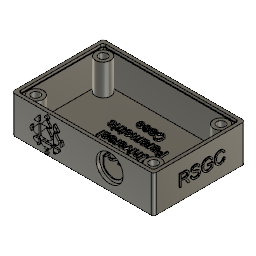
ACESUniversalST1StripboardCase v4 (Autodesk Fusion 360 design; units mm, degrees)
Autodesk Fusion 360 part; units mm, degrees
note: some values were not read from the file. Set by a fixed rule: which sketch regions a step uses.
sketch "PCB" plane through (0, 0, 0) normal (0, 0, 1) x (1, 0, 0)
  line L0 (0, 0) -> (80, 0)
  line L1 (80, 0) -> (80, 50)
  line L2 (80, 50) -> (0, 50)
  line L3 (0, 50) -> (0, 0)
  line L4 (-0.25, -0.25) -> (80.25, -0.25)
  line L5 (80.25, -0.25) -> (80.25, 50.25)
  line L6 (80.25, 50.25) -> (-0.25, 50.25)
  line L7 (-0.25, 50.25) -> (-0.25, -0.25)
  line L8 (79.75, 0.25) -> (79.75, 49.75)
  line L9 (79.75, 49.75) -> (0.25, 49.75)
  line L10 (0.25, 49.75) -> (0.25, 0.25)
  line L11 (0.25, 0.25) -> (79.75, 0.25)
  line L12 (82.25, 52.25) -> (-2.25, 52.25)
  line L13 (-2.25, 52.25) -> (-2.25, -2.25)
  line L14 (-2.25, -2.25) -> (82.25, -2.25)
  line L15 (82.25, -2.25) -> (82.25, 52.25)
  dimension "d7" = 80
  dimension "d8" = 50
  dimension "d30" = 0.25
  dimension "d32" = 2.25
  constraint horizontal L0
  constraint vertical L1
  constraint horizontal L2
  constraint vertical L3
  constraint coincident L0.start L3.end
  measures "d7" distance of L0.start L0.end
  measures "d8" distance of L0.start L2.end
sketch "Piers" plane through (0, 0, 0) normal (0, 0, 1) x (1, 0, 0)
  line L0 (80, 50) -> (0, 50)
  circle A0 centre (5, 45) radius 4.5
  circle A1 centre (5, 45) radius 2.5
  line L1 (0, 50) -> (0, 0)
  line L2 (0, 0) -> (80, 0)
  circle A2 centre (5, 5) radius 4.5
  circle A3 centre (5, 5) radius 2.5
  line L3 (80, 0) -> (80, 50)
  circle A4 centre (75, 45) radius 4.5
  circle A5 centre (75, 45) radius 2.5
  circle A6 centre (75, 5) radius 4.5
  circle A7 centre (75, 5) radius 2.5
  point P0 (5, 45)
  point P1 (0, 50)
  point P2 (5, 5)
  point P3 (75, 45)
  point P4 (75, 5)
  point P5 (75, 5)
  dimension "d10" = 5
  dimension "d11" = 5
  dimension "d13" = 9
  dimension "d15" = 5
  dimension "d16" = 5
  dimension "d17" = 5
  dimension "d18" = 9
  dimension "d19" = 5
  dimension "d20" = 5
  dimension "d21" = 5
  dimension "d22" = 9
  dimension "d23" = 5
  dimension "d24" = 5
  dimension "d25" = 5
  dimension "d26" = 9
  dimension "d27" = 5
  constraint coincident P0 A0.centre
  constraint coincident P2 A2.centre
  constraint coincident P3 A4.centre
  constraint coincident P5 P4
  constraint concentric A6 A7
  measures "d10" horizontal distance of P0 L0.end
  measures "d11" distance of P0 L0
  measures "d13" diameter of A0
  measures "d15" diameter of A1
  measures "d16" distance of P2 L1
  measures "d17" distance of P2 L2
  measures "d18" diameter of A2
  measures "d19" diameter of A3
  measures "d20" distance of P3 L3
  measures "d21" distance of L0 P3
  measures "d22" diameter of A4
  measures "d23" diameter of A5
  measures "d24" distance of L3 P5
  measures "d25" distance of L2 P5
  measures "d26" diameter of A6
  measures "d27" diameter of A7
extrude "Extrude1" add sketch "Piers" along normal blind 20.4 contours A4 makes body 1
extrude "Extrude2" add sketch "Piers" along normal blind 13 contours A5 bodies 1
extrude "Extrude3" add sketch "Piers" along normal blind 13 separate body contours A7 makes body 2
extrude "Extrude4" add sketch "Piers" along normal blind 20.4 contours A6 bodies 2
extrude "Extrude5" add sketch "Piers" along normal blind 13 separate body contours A3 makes body 3
extrude "Extrude6" add sketch "Piers" along normal blind 20.4 contours A2 bodies 3
extrude "Extrude7" add sketch "Piers" along normal blind 13 separate body contours A1 makes body 4
extrude "Extrude8" add sketch "Piers" along normal blind 20.4 contours A0 bodies 4
extrude "Extrude9" cut sketch "PCB" along normal blind 2 contours L8 L9 L10 L11 bodies 1 2 3 4
extrude "Extrude10" add sketch "PCB" along normal blind 2 contours L8 L9 L10 L11 bodies 1 2 3 4
extrude "Extrude11" add sketch "PCB" along normal blind 20.4 contours L0 L1 L2 L3 bodies 1
extrude "Extrude12" add sketch "PCB" along normal blind 20.4 contours L4 L5 L6 L7 bodies 1
extrude "Extrude13" add sketch "PCB" along normal blind 22 contours L12 L13 L14 L15 bodies 1
fillet "Fillet1" radius 1.5 4 edges at (82.25, -2.25, 11) (-2.25, -2.25, 11) (82.25, 52.25, 11) (-2.25, 52.25, 11) on bodies 1
fillet "Fillet2" radius 1.5 1 edges at (80.25, -0.25, 21.2) on bodies 1
fillet "Fillet3" radius 1.5 1 edges at (-0.25, 50.25, 21.2) on bodies 1
fillet "Fillet4" radius 1.5 1 edges at (-0.25, -0.25, 21.2) on bodies 1
fillet "Fillet5" radius 1.5 1 edges at (80.25, 50.25, 21.2) on bodies 1
sketch "SchurterPJ" plane through (0, -2.25, 0) normal (0, -1, 0) x (1, 0, 0)
  line L0 (-0.75, 22) -> (-0.75, 0)
  line L1 (-0.75, 0) -> (80.75, 0)
  line L2 (80.75, 0) -> (80.75, 22)
  line L3 (80.75, 22) -> (-0.75, 22)
  circle A0 centre (56.0888, 11.8801) radius 8
  circle A1 centre (56.0888, 11.8801) radius 6.4
  line L4 (50.1888, 9.4002) -> (50.1888, 14.36)
  line L5 (61.9888, 14.36) -> (61.9888, 9.4002)
  line L6 (61.9888, 9.4002) -> (50.1888, 14.36) construction
  line L7 (50.1888, 9.4002) -> (61.9888, 14.36) construction
  point P0 (56.0888, 11.8801)
  dimension "d84" = 16
  dimension "d85" = 12.8
  dimension "d86" = 11.8
  constraint concentric A0 A1
  constraint parallel L4 L5
  constraint coincident L6 P0
  constraint coincident L7 P0
  constraint coincident A1 L5.end
  constraint coincident P0 A0.centre
  measures "d84" diameter of A0
  measures "d85" diameter of A1
  measures "d86" distance of L4.end L5.start
extrude "Extrude16" cut sketch "SchurterPJ" against normal blind 4 contours A1 L4 L5 bodies 1
extrude "Extrude17" cut sketch "SchurterPJ" against normal blind 2 contours A0 bodies 1
extrude "Extrude18" cut sketch "SchurterPJ" against normal blind 2 contours A1 L4 bodies 1
extrude "Extrude19" cut sketch "SchurterPJ" against normal blind 2 contours A1 L5 bodies 1
sketch "RSGC" plane through (82.25, 0, 0) normal (1, 0, 0) x (0, 1, 0)
  line L0 (50.75, 0) -> (50.75, 22)
  line L1 (50.75, 22) -> (-0.75, 22)
  line L2 (-0.75, 22) -> (-0.75, 0)
  line L3 (-0.75, 0) -> (50.75, 0)
  line L4 (6.6478, 4.3711) -> (45.8969, 4.3711) construction
  line L5 (45.8969, 4.3711) -> (45.8969, 17.8488) construction
  line L6 (45.8969, 17.8488) -> (6.6478, 17.8488) construction
  line L7 (6.6478, 17.8488) -> (6.6478, 4.3711) construction
  dimension "d101" = 7
  text T0 "RSGC" font "Arial" height 7 align centre middle in box 39.2491 x 13.4777 at (6.6478, 4.3711) x (1, 0) y (0, 1) spacing 1
extrude "Extrude23" add sketch "RSGC" along normal blind 0.5 text T0 bodies 1
sketch "ACES" plane through (-2.25, 0, 0) normal (-1, 0, 0) x (0, -1, 0)
  line L0 (-50.75, 22) -> (-50.75, 0)
  line L1 (-50.75, 0) -> (0.75, 0)
  line L2 (0.75, 0) -> (0.75, 22)
  line L3 (0.75, 22) -> (-50.75, 22)
  line L4 (-44.8392, 4.4236) -> (-4.5213, 4.4236) construction
  line L5 (-4.5213, 4.4236) -> (-4.5213, 18.3404) construction
  line L6 (-4.5213, 18.3404) -> (-44.8392, 18.3404) construction
  line L7 (-44.8392, 18.3404) -> (-44.8392, 4.4236) construction
  dimension "d105" = 7
  text T0 "ACES" font "Arial" height 7 align centre middle in box 40.3179 x 13.9168 at (-44.8392, 4.4236) x (1, 0) y (0, 1) spacing 1
extrude "Extrude24" add sketch "ACES" along normal blind 0.5 text T0 bodies 1
sketch "Stripboard" plane through (0, 52.25, 0) normal (0, 1, 0) x (-1, 0, 0)
  line L0 (0.75, 0) -> (0.75, 22)
  line L1 (0.75, 22) -> (-80.75, 22)
  line L2 (-80.75, 22) -> (-80.75, 0)
  line L3 (-80.75, 0) -> (0.75, 0)
  line L4 (-75.2707, 4.2089) -> (-2.7407, 4.2089) construction
  line L5 (-2.7407, 4.2089) -> (-2.7407, 18.6953) construction
  line L6 (-2.7407, 18.6953) -> (-75.2707, 18.6953) construction
  line L7 (-75.2707, 18.6953) -> (-75.2707, 4.2089) construction
  dimension "d108" = 7
  text T0 "Stripboard" font "Arial" height 7 align centre middle in box 72.53 x 14.4864 at (-75.2707, 4.2089) x (1, 0) y (0, 1) spacing 1
extrude "Extrude25" add sketch "Stripboard" along normal blind 0.5 text T0 bodies 1
sketch "ACESLogo" plane through (0, -2.25, 0) normal (0, -1, 0) x (1, 0, 0)
  line L0 (-0.75, 22) -> (-0.75, 0)
  line L1 (-0.75, 0) -> (80.75, 0)
  line L2 (80.75, 0) -> (80.75, 22)
  line L3 (80.75, 22) -> (-0.75, 22)
  circle A0 centre (56.0888, 11.8801) radius 8
  arc A1 (18.9448, 9.0125) -> (17.9359, 8.8538) centre (17.8817, 12.4835) cw
  spline S0 degree 3 poles (17.9359, 8.8538) (17.1335, 8.9002) (16.4759, 9.5075) (16.366, 10.3037) knots 1 1 1 1 2 2 2 2
  arc A2 (16.366, 10.3037) -> (16.8211, 11.6936) centre (18.2653, 10.4513) cw
  spline S1 degree 3 poles (16.8211, 11.6936) (17.5549, 12.5932) (18.2992, 13.4857) (19.033, 14.3889) knots 3 3 3 3 4 4 4 4
  spline S2 degree 3 poles (19.033, 14.3889) (19.193, 14.597) (19.4912, 14.6364) (19.6997, 14.4771) knots 4 4 4 4 5 5 5 5
  arc A3 (19.6997, 14.4771) -> (19.7879, 14.3889) centre (19.4528, 14.1419) cw
  spline S3 degree 3 poles (19.7879, 14.3889) (20.2289, 13.8279) (20.6981, 13.2952) (21.1497, 12.7449) knots 6 6 6 6 7 7 7 7
  arc A4 (21.1497, 12.7449) -> (22.1657, 11.482) centre (10.8021, 3.3805) cw
  spline S4 degree 3 poles (22.1657, 11.482) (22.695, 10.7422) (22.5262, 9.7137) (21.7882, 9.1819) knots 8 8 8 8 9 9 9 9
  arc A5 (21.7882, 9.1819) -> (21.2026, 8.9173) centre (20.8109, 10.5647) cw
  arc A6 (21.2026, 8.9173) -> (20.0702, 8.9737) centre (20.7508, 11.2409) cw
  spline S5 degree 3 poles (20.0702, 8.9737) (20.0067, 8.9737) (19.922, 9.0549) (19.8373, 8.949) (19.9044, 8.8749) (19.9255, 8.8114) knots 11 11 11 11 12 12 13 13 13 13
  arc A7 (19.9255, 8.8114) -> (20.2889, 8.1659) centre (23.5074, 10.4024) ccw
  spline S6 degree 3 poles (20.2889, 8.1659) (20.3348, 8.0953) (20.3947, 8.0212) (20.2889, 7.8378) (20.2007, 7.8554) (20.1125, 7.8554) knots 14 14 14 14 15 15 16 16 16 16
  line L4 (20.1125, 7.8554) -> (18.7014, 7.8554)
  arc A8 (18.7014, 7.8554) -> (18.5215, 7.9366) centre (18.6835, 8.0557) cw
  spline S7 degree 3 poles (18.5215, 7.9366) (18.4721, 8.0106) (18.5215, 8.0706) (18.5497, 8.1306) knots 18 18 18 18 19 19 19 19
  arc A9 (18.5497, 8.1306) -> (18.9448, 9.0125) centre (16.2293, 9.6996) ccw
  arc A10 (19.862, 4.8674) -> (20.2501, 4.0101) centre (22.6563, 5.6158) ccw
  arc A11 (20.2501, 4.0101) -> (20.3171, 3.9114) centre (19.4824, 3.4171) cw
  spline S8 degree 3 poles (20.3171, 3.9114) (20.3585, 3.843) (20.3367, 3.7541) (20.2684, 3.7127) knots 2 2 2 2 3 3 3 3
  spline S9 degree 3 poles (20.2684, 3.7127) (20.267, 3.7119) (20.2656, 3.7111) (20.2642, 3.7103) knots 3 3 3 3 4 4 4 4
  arc A12 (20.2642, 3.7103) -> (20.1795, 3.6891) centre (20.1938, 3.8118) cw
  line L5 (20.1795, 3.6891) -> (18.6308, 3.6891)
  spline S10 degree 3 poles (18.6308, 3.6891) (18.4862, 3.6891) (18.4297, 3.802) (18.5074, 3.929) knots 6 6 6 6 7 7 7 7
  arc A13 (18.5074, 3.929) -> (18.9025, 4.7016) centre (15.4234, 5.9935) ccw
  spline S11 degree 3 poles (18.9025, 4.7016) (18.9201, 4.751) (18.9519, 4.8074) (18.8531, 4.878) (18.8213, 4.8427) (18.779, 4.8215) knots 8 8 8 8 9 9 10 10 10 10
  arc A14 (18.779, 4.8215) -> (17.3467, 4.8427) centre (18.0946, 6.9768) cw
  spline S12 degree 3 poles (17.3467, 4.8427) (16.7529, 5.0971) (16.3626, 5.675) (16.3484, 6.3208) knots 11 11 11 11 12 12 12 12
  arc A15 (16.3484, 6.3208) -> (16.4083, 6.8077) centre (18.2321, 6.3359) cw
  spline S13 degree 3 poles (16.4083, 6.8077) (16.4227, 6.8898) (16.4982, 6.9469) (16.5812, 6.9382) knots 13 13 13 13 14 14 14 14
  line L6 (16.5812, 6.9382) -> (22.1445, 6.9382)
  spline S14 degree 3 poles (22.1445, 6.9382) (22.3032, 6.9382) (22.3738, 6.8853) (22.4056, 6.7406) knots 15 15 15 15 16 16 16 16
  spline S15 degree 3 poles (22.4056, 6.7406) (22.6249, 5.8696) (22.0966, 4.9858) (21.2256, 4.7664) knots 16 16 16 16 17 17 17 17
  line L7 (21.2256, 4.7664) -> (21.2202, 4.7651)
  line L8 (21.2202, 4.7651) -> (21.1673, 4.7651)
  arc A16 (21.1673, 4.7651) -> (19.862, 4.8674) centre (20.7187, 7.4191) cw
  spline S16 degree 3 poles (14.5139, 9.0125) (14.2846, 8.9561) (14.0659, 8.9102) (13.8472, 8.8749) knots 0 0 0 0 1 1 1 1
  spline S17 degree 3 poles (13.8472, 8.8749) (12.9414, 8.7275) (12.0877, 9.3423) (11.9402, 10.248) (11.8627, 10.7242) (11.9961, 11.2106) (12.3055, 11.5808) knots 1 1 1 1 2 2 2 3 3 3 3
  spline S18 degree 3 poles (12.3055, 11.5808) (12.7394, 12.1417) (13.2016, 12.6779) (13.6461, 13.2247) knots 3 3 3 3 4 4 4 4
  line L9 (13.6461, 13.2247) -> (14.6056, 14.3959)
  arc A17 (14.6056, 14.3959) -> (14.9584, 14.5723) centre (14.9478, 14.1526) cw
  spline S19 degree 3 poles (14.9584, 14.5723) (15.046, 14.5763) (15.1202, 14.5085) (15.1242, 14.4209) knots 6 6 6 6 7 7 7 7
  line L10 (15.1242, 14.4209) -> (15.1242, 14.4206)
  line L11 (15.1242, 14.4206) -> (15.1242, 8.0142)
  spline S20 degree 3 poles (15.1242, 8.0142) (15.144, 7.9237) (15.0874, 7.8341) (14.9972, 7.8131) knots 9 9 9 9 10 10 10 10
  line L12 (14.9972, 7.8131) -> (14.2423, 7.8131)
  arc A18 (14.2423, 7.8131) -> (14.0518, 7.9083) centre (14.2177, 8.002) cw
  spline S21 degree 3 poles (14.0518, 7.9083) (14.0059, 7.9754) (14.0518, 8.0318) (14.0871, 8.0847) knots 12 12 12 12 13 13 13 13
  arc A19 (14.0871, 8.0847) -> (14.5139, 9.0125) centre (11.5121, 9.8315) ccw
  line L13 (23.7002, 11.2068) -> (23.7002, 14.3077)
  spline S22 degree 3 poles (23.7002, 14.3077) (23.7002, 14.3994) (23.6614, 14.5159) (23.7814, 14.5582) knots 1 1 1 1 2 2 2 2
  arc A20 (23.7814, 14.5582) -> (24.1059, 14.4876) centre (23.8827, 14.2424) cw
  arc A21 (24.1059, 14.4876) -> (24.4305, 14.1102) centre (22.3461, 12.6463) cw
  spline S23 degree 3 poles (24.4305, 14.1102) (25.1184, 13.2811) (25.8169, 12.4556) (26.4837, 11.609) knots 4 4 4 4 5 5 5 5
  spline S24 degree 3 poles (26.4837, 11.609) (27.0909, 10.9209) (27.0253, 9.8709) (26.3372, 9.2637) (25.9609, 8.9316) (25.4545, 8.7874) (24.9597, 8.8714) knots 5 5 5 5 6 6 6 7 7 7 7
  spline S25 degree 3 poles (24.9597, 8.8714) (24.7692, 8.8996) (24.5857, 8.9314) (24.3988, 8.9772) knots 7 7 7 7 8 8 8 8
  spline S26 degree 3 poles (24.3988, 8.9772) (24.3705, 8.9772) (24.3458, 9.0161) (24.2894, 8.9384) (24.3176, 8.9243) (24.3176, 8.8926) knots 8 8 8 8 9 9 10 10 10 10
  arc A22 (24.3176, 8.8926) -> (24.6457, 8.187) centre (27.442, 9.9164) ccw
  spline S27 degree 3 poles (24.6457, 8.187) (24.7021, 8.0882) (24.815, 7.9965) (24.681, 7.7496) (24.5399, 7.8025) (24.4305, 7.799) knots 11 11 11 11 12 12 13 13 13 13
  line L14 (24.4305, 7.799) -> (23.9013, 7.799)
  spline S28 degree 3 poles (23.9013, 7.799) (23.7249, 7.799) (23.6967, 7.8342) (23.6967, 8.0001) knots 14 14 14 14 15 15 15 15
  line L15 (23.6967, 8.0001) -> (23.7002, 11.2068)
  line L16 (21.8023, 15.5036) -> (20.4723, 15.5036)
  spline S29 degree 3 poles (20.4723, 15.5036) (19.9679, 15.5036) (19.4599, 15.4789) (18.9554, 15.5036) knots 1 1 1 1 2 2 2 2
  line L17 (18.9554, 15.5036) -> (16.8952, 15.5036)
  arc A23 (16.8952, 15.5036) -> (16.7223, 15.5918) centre (16.8776, 15.6827) cw
  ellipse E0 centre (16.8568, 15.657) end of major axis (16.8885, 15.804) minor radius 0.1488 (16.7611, 15.7717) -> (16.7223, 15.5918) ccw
  arc A24 (16.7611, 15.7717) -> (19.033, 18.5305) centre (514.2406, -391.6025) cw
  spline S30 degree 3 poles (19.033, 18.5305) (19.1707, 18.7375) (19.4498, 18.7943) (19.6574, 18.6575) knots 6 6 6 6 7 7 7 7
  arc A25 (19.6574, 18.6575) -> (19.7985, 18.5093) centre (19.42, 18.2901) cw
  spline S31 degree 3 poles (19.7985, 18.5093) (20.1125, 18.1177) (20.4406, 17.7367) (20.7616, 17.3487) knots 8 8 8 8 9 9 9 9
  line L18 (20.7616, 17.3487) -> (21.8199, 16.054)
  spline S32 degree 3 poles (21.8199, 16.054) (21.8976, 15.9587) (21.9716, 15.8635) (22.0528, 15.7753) knots 10 10 10 10 11 11 11 11
  ellipse E1 centre (21.9602, 15.6624) end of major axis (21.9286, 15.8059) minor radius 0.1453 (22.0916, 15.5989) -> (22.0528, 15.7753) ccw
  spline S33 degree 3 poles (22.0916, 15.5989) (22.0643, 15.5318) (21.9934, 15.4934) (21.9223, 15.5072) knots 12 12 12 12 13 13 13 13
  arc A26 (21.9223, 15.5072) -> (21.8023, 15.5036) centre (21.8725, 15.1579) ccw
  arc A27 (24.3423, 4.8603) -> (24.748, 3.9996) centre (27.4138, 5.782) ccw
  spline S34 degree 3 poles (24.748, 3.9996) (24.7903, 3.9325) (24.8397, 3.869) (24.748, 3.6926) (24.6669, 3.7138) (24.5963, 3.7138) knots 1 1 1 1 2 2 3 3 3 3
  line L19 (24.5963, 3.7138) -> (23.919, 3.7138)
  spline S35 degree 3 poles (23.919, 3.7138) (23.7849, 3.7138) (23.732, 3.7703) (23.732, 3.9043) knots 4 4 4 4 5 5 5 5
  line L20 (23.732, 3.9043) -> (23.732, 6.7547)
  spline S36 degree 3 poles (23.732, 6.7547) (23.732, 6.8853) (23.7884, 6.9523) (23.919, 6.9523) knots 6 6 6 6 7 7 7 7
  line L21 (23.919, 6.9523) -> (26.6848, 6.9523)
  spline S37 degree 3 poles (26.6848, 6.9523) (26.7676, 6.9636) (26.8454, 6.9102) (26.8647, 6.8288) knots 8 8 8 8 9 9 9 9
  spline S38 degree 3 poles (26.8647, 6.8288) (27.1112, 5.957) (26.6043, 5.0505) (25.7325, 4.804) knots 9 9 9 9 10 10 10 10
  line L22 (25.7325, 4.804) -> (25.7323, 4.8039)
  arc A28 (25.7323, 4.8039) -> (25.5029, 4.758) centre (25.2724, 6.5069) cw
  arc A29 (25.5029, 4.758) -> (24.4446, 4.878) centre (25.2859, 7.5719) cw
  line L23 (24.4446, 4.878) -> (24.3846, 4.878)
  line L24 (24.3846, 4.878) -> (24.3423, 4.8603)
  arc A30 (14.5104, 4.8639) -> (13.5226, 4.7192) centre (13.4801, 8.4549) cw
  spline S39 degree 3 poles (13.5226, 4.7192) (12.9343, 4.7273) (12.3955, 5.0506) (12.1115, 5.5659) knots 1 1 1 1 2 2 2 2
  arc A31 (12.1115, 5.5659) -> (11.9669, 6.7547) centre (13.4646, 6.3337) cw
  spline S40 degree 3 poles (11.9669, 6.7547) (11.9862, 6.8526) (12.0755, 6.9207) (12.175, 6.9135) knots 3 3 3 3 4 4 4 4
  line L25 (12.175, 6.9135) -> (14.8949, 6.9135)
  spline S41 degree 3 poles (14.8949, 6.9135) (15.0748, 6.9135) (15.1066, 6.8747) (15.1066, 6.6877) knots 5 5 5 5 6 6 6 6
  line L26 (15.1066, 6.6877) -> (15.1066, 3.8973)
  spline S42 degree 3 poles (15.1066, 3.8973) (15.1066, 3.7456) (15.0572, 3.6891) (14.902, 3.6891) knots 7 7 7 7 8 8 8 8
  line L27 (14.902, 3.6891) -> (14.2493, 3.6891)
  arc A32 (14.2493, 3.6891) -> (14.0518, 3.7703) centre (14.2137, 3.8834) cw
  spline S43 degree 3 poles (14.0518, 3.7703) (14.0024, 3.8514) (14.0518, 3.9043) (14.0906, 3.9643) knots 10 10 10 10 11 11 11 11
  arc A33 (14.0906, 3.9643) -> (14.5104, 4.8639) centre (11.6628, 5.645) ccw
  line L28 (23.7285, 17.0982) -> (23.7285, 18.5093)
  spline S44 degree 3 poles (23.7285, 18.5093) (23.7285, 18.6963) (23.8167, 18.7739) (24.0248, 18.7139) knots 1 1 1 1 2 2 2 2
  arc A34 (24.0248, 18.7139) -> (24.2329, 18.5728) centre (23.902, 18.3088) cw
  line L29 (24.2329, 18.5728) -> (25.2913, 17.2746)
  line L30 (25.2913, 17.2746) -> (26.4696, 15.8635)
  arc A35 (26.4696, 15.8635) -> (26.5613, 15.7435) centre (26.0428, 15.4421) cw
  spline S45 degree 3 poles (26.5613, 15.7435) (26.6007, 15.6832) (26.5837, 15.6023) (26.5234, 15.5629) knots 6 6 6 6 7 7 7 7
  ellipse E2 centre (26.4292, 15.6661) end of major axis (26.5726, 15.6299) minor radius 0.1252 (26.5189, 15.5601) -> (26.5234, 15.5629) ccw
  arc A36 (26.5189, 15.5601) -> (26.4449, 15.5389) centre (26.4426, 15.6871) cw
  line L31 (26.4449, 15.5389) -> (23.8625, 15.5389)
  spline S46 degree 3 poles (23.8625, 15.5389) (23.7355, 15.5389) (23.7249, 15.6271) (23.7249, 15.7259) knots 10 10 10 10 11 11 11 11
  line L32 (23.7249, 15.7259) -> (23.7249, 17.0982)
  line L33 (23.7249, 17.0982) -> (23.7285, 17.0982)
  spline S47 degree 3 poles (15.096, 17.458) (15.1278, 17.0559) (15.0784, 16.5796) (15.1172, 16.1069) knots 0 0 0 0 1 1 1 1
  line L34 (15.1172, 16.1069) -> (15.1172, 15.6589)
  spline S48 degree 3 poles (15.1172, 15.6589) (15.1232, 15.5753) (15.0604, 15.5027) (14.9768, 15.4966) knots 2 2 2 2 3 3 3 3
  line L35 (14.9768, 15.4966) -> (14.9761, 15.4966)
  line L36 (14.9761, 15.4966) -> (13.3674, 15.4966)
  line L37 (13.3674, 15.4966) -> (12.4149, 15.4966)
  spline S49 degree 3 poles (12.4149, 15.4966) (12.3393, 15.4884) (12.2715, 15.5431) (12.2633, 15.6186) knots 6 6 6 6 7 7 7 7
  line L38 (12.2633, 15.6186) -> (12.2632, 15.6201)
  arc A37 (12.2632, 15.6201) -> (12.3091, 15.7365) centre (12.4075, 15.6305) cw
  spline S50 degree 3 poles (12.3091, 15.7365) (12.6618, 16.1633) (13.0146, 16.5902) (13.3674, 17.01) knots 9 9 9 9 10 10 10 10
  line L39 (13.3674, 17.01) -> (14.2917, 18.1989)
  spline S51 degree 3 poles (14.2917, 18.1989) (14.394, 18.3259) (14.4998, 18.4564) (14.6056, 18.5799) knots 11 11 11 11 12 12 12 12
  arc A38 (14.6056, 18.5799) -> (14.909, 18.721) centre (14.9246, 18.2909) cw
  spline S52 degree 3 poles (14.909, 18.721) (14.9941, 18.7316) (15.0717, 18.6713) (15.0823, 18.5862) (15.084, 18.5724) (15.0839, 18.5584) (15.0819, 18.5446) knots 13 13 13 13 14 14 14 15 15 15 15
  spline S53 degree 3 poles (15.0819, 18.5446) (15.0925, 18.2059) (15.096, 17.8672) (15.096, 17.458) knots 15 15 15 15 16 16 16 16
  line L40 (27.7784, 10.6565) -> (27.7784, 12.1276)
  spline S54 degree 3 poles (27.7784, 12.1276) (27.7784, 12.2087) (27.7784, 12.2863) (27.8666, 12.3181) knots 1 1 1 1 2 2 2 2
  spline S55 degree 3 poles (27.8666, 12.3181) (27.9344, 12.3499) (28.0153, 12.3274) (28.0571, 12.2651) knots 2 2 2 2 3 3 3 3
  spline S56 degree 3 poles (28.0571, 12.2651) (28.2617, 11.9935) (28.5121, 11.7536) (28.6921, 11.4608) knots 3 3 3 3 4 4 4 4
  spline S57 degree 3 poles (28.6921, 11.4608) (29.0878, 10.8976) (29.0962, 10.1489) (28.7132, 9.577) knots 4 4 4 4 5 5 5 5
  arc A39 (28.7132, 9.577) -> (28.05, 9.0196) centre (27.2815, 10.6073) cw
  spline S58 degree 3 poles (28.05, 9.0196) (27.8736, 8.9279) (27.7713, 8.9984) (27.7713, 9.1995) knots 6 6 6 6 7 7 7 7
  line L41 (27.7713, 9.1995) -> (27.7713, 10.6565)
  line L42 (27.7713, 10.6565) -> (27.7784, 10.6565)
  line L43 (11.0214, 10.6353) -> (11.0214, 9.1889)
  ellipse E3 centre (9.7021, 11.0867) end of major axis (8.4539, 13.1795) minor radius 0.4973 (10.7533, 9.0196) -> (11.0214, 9.1889) ccw
  spline S59 degree 3 poles (10.7533, 9.0196) (10.2762, 9.2397) (9.9355, 9.6777) (9.8396, 10.1943) knots 2 2 2 2 3 3 3 3
  ellipse E4 centre (11.5641, 10.4916) end of major axis (12.0331, 12.1844) minor radius 1.7485 (10.2383, 11.6337) -> (9.8396, 10.1943) ccw
  spline S60 degree 3 poles (10.2383, 11.6337) (10.4111, 11.8489) (10.5804, 12.0464) (10.7639, 12.2722) knots 4 4 4 4 5 5 5 5
  ellipse E5 centre (10.8827, 12.1875) end of major axis (11.0242, 12.2271) minor radius 0.1453 (10.9403, 12.3216) -> (10.7639, 12.2722) ccw
  spline S61 degree 3 poles (10.9403, 12.3216) (11.0179, 12.2934) (11.0355, 12.2334) (11.0355, 12.1558) knots 6 6 6 6 7 7 7 7
  spline S62 degree 3 poles (11.0355, 12.1558) (11.0179, 11.6513) (11.0214, 11.1504) (11.0214, 10.6353) knots 7 7 7 7 8 8 8 8
  line L44 (19.3964, 19.5888) -> (18.338, 19.5888)
  spline S63 degree 3 poles (18.338, 19.5888) (18.2569, 19.5888) (18.1863, 19.5888) (18.1087, 19.7723) (18.1475, 19.8146) (18.204, 19.871) knots 1 1 1 1 2 2 3 3 3 3
  line L45 (18.204, 19.871) -> (19.0647, 20.9294)
  spline S64 degree 3 poles (19.0647, 20.9294) (19.2324, 21.1162) (19.5197, 21.132) (19.7068, 20.9646) knots 4 4 4 4 5 5 5 5
  ellipse E6 centre (19.4906, 20.7133) end of major axis (19.8199, 20.6741) minor radius 0.3315 (19.7421, 20.9294) -> (19.7068, 20.9646) ccw
  spline S65 degree 3 poles (19.7421, 20.9294) (20.0419, 20.5766) (20.3277, 20.2238) (20.6205, 19.8534) knots 6 6 6 6 7 7 7 7
  spline S66 degree 3 poles (20.6205, 19.8534) (20.6664, 19.8005) (20.7157, 19.7476) (20.6699, 19.6664) knots 7 7 7 7 8 8 8 8
  ellipse E7 centre (20.5127, 19.7561) end of major axis (20.678, 19.8325) minor radius 0.1804 (20.4794, 19.5782) -> (20.6699, 19.6664) ccw
  line L46 (20.4794, 19.5782) -> (19.3964, 19.5888)
  line L47 (19.414, 1.3431) -> (18.6414, 1.3431)
  arc A40 (18.6414, 1.3431) -> (18.4862, 1.4137) centre (18.6157, 1.4926) cw
  arc A41 (18.4862, 1.4137) -> (18.5109, 1.5971) centre (18.6432, 1.4859) cw
  arc A42 (18.5109, 1.5971) -> (18.9413, 2.4932) centre (16.2025, 3.2573) ccw
  line L48 (18.9413, 2.4932) -> (18.9413, 2.5214)
  spline S67 degree 3 poles (18.9413, 2.5214) (19.0118, 2.8742) (19.0118, 2.8742) (19.3576, 2.8742) knots 5 5 5 5 6 6 6 6
  line L49 (19.3576, 2.8742) -> (19.6292, 2.8742)
  spline S68 degree 3 poles (19.6292, 2.8742) (19.7167, 2.8892) (19.8001, 2.831) (19.8162, 2.7437) knots 7 7 7 7 8 8 8 8
  ellipse E8 centre (19.7718, 2.7331) end of major axis (19.7718, 2.7788) minor radius 0.0456 (19.8162, 2.7225) -> (19.8162, 2.7437) ccw
  arc A43 (19.8162, 2.7225) -> (20.2889, 1.6289) centre (22.142, 3.0789) ccw
  arc A44 (20.2889, 1.6289) -> (20.3277, 1.4031) centre (20.1045, 1.481) cw
  spline S69 degree 3 poles (20.3277, 1.4031) (20.2959, 1.329) (20.2113, 1.3431) (20.1407, 1.3431) knots 11 11 11 11 12 12 12 12
  line L50 (20.1407, 1.3431) -> (19.414, 1.3431)
extrude "Extrude27" add sketch "ACESLogo" along normal blind 1 contours A1 S0 A2 S1 S2 A3 S3 A4 S4 A5 A6 S5 A7 S6 L4 A8 S7 A9 | A10 A11 S8 S9 A12 L5 S10 A13 S11 A14 S12 A15 S13 L6 S14 S15 L7 L8 A16 | S16 S17 S18 L9 A17 S19 L11 S20 L12 A18 S21 A19 | L13 S22 A20 A21 S23 S24 S25 S26 A22 S27 L14 S28 L15 | L16 S29 L17 A23 E0 A24 S30 A25 S31 L18 S32 E1 S33 A26 | A27 S34 L19 S35 L20 S36 L21 S37 S38 A28 A29 L23 L24 | A30 S39 A31 S40 L25 S41 L26 S42 L27 A32 S43 A33 | L28 S44 A34 L29 L30 A35 S45 E2 A36 L31 S46 L32 L33 | S47 L34 S48 L36 L37 S49 A37 S50 L39 S51 A38 S52 S53 | L40 S54 S55 S56 S57 A39 S58 L41 L42 | L43 E3 S59 E4 S60 E5 S61 S62 | L44 S63 L45 S64 E6 S65 S66 E7 L46 | L47 A40 A41 A42 L48 S67 L49 S68 E8 A43 A44 S69 L50 bodies 1
sketch "Sketch21" plane through (0, 0, 2) normal (0, 0, 1) x (-1, 0, 0)
  circle A0 centre (-5, -5) radius 4.5
  circle A1 centre (-75, -45) radius 4.5
  circle A2 centre (-75, -5) radius 4.5
  circle A3 centre (-5, -45) radius 4.5
  line L0 (-0.25, -0.25) -> (-79.75, -0.25)
  line L1 (-79.75, -0.25) -> (-79.75, -49.75)
  line L2 (-79.75, -49.75) -> (-0.25, -49.75)
  line L3 (-0.25, -49.75) -> (-0.25, -0.25)
  line L4 (-64.3759, -45.9893) -> (-14.8917, -45.9893) construction
  line L5 (-14.8917, -45.9893) -> (-14.8917, -6.2806) construction
  line L6 (-14.8917, -6.2806) -> (-64.3759, -6.2806) construction
  line L7 (-64.3759, -6.2806) -> (-64.3759, -45.9893) construction
  dimension "d127" = 5
  text T0 "ACES\nUniversal\nParametric\nCase" font "Arial" height 5 align centre middle in box 49.4842 x 39.7087 at (-64.3759, -45.9893) x (1, 0) y (0, 1) spacing 1
extrude "Extrude34" add sketch "Sketch21" along normal blind 1 text T0 bodies 1
extrude "Extrude32" [suppressed]
extrude "Extrude30" [suppressed]
extrude "Extrude29" [suppressed]
extrude "Extrude28" [suppressed]
extrude "Extrude26" [suppressed]
extrude "Extrude22" [suppressed]
extrude "Extrude21" [suppressed]
equation "pcbWidth = 80 mm"
equation "pcbHeight = 50 mm"
equation "d7 = pcbWidth"
equation "d8 = pcbHeight"
equation "pierCornerOffset = 5 mm"
equation "d10 = pierCornerOffset"
equation "d11 = pierCornerOffset"
equation "pierOuterDiameter = 9 mm"
equation "d13 = pierOuterDiameter"
equation "pierInnerDiameter = 5 mm"
equation "d15 = pierInnerDiameter"
equation "d16 = pierCornerOffset"
equation "d17 = pierCornerOffset"
equation "d18 = pierOuterDiameter"
equation "d19 = pierInnerDiameter"
equation "d20 = pierCornerOffset"
equation "d21 = pierCornerOffset"
equation "d22 = pierOuterDiameter"
equation "d23 = pierInnerDiameter"
equation "d24 = pierCornerOffset"
equation "d25 = pierCornerOffset"
equation "d26 = pierOuterDiameter"
equation "d27 = pierInnerDiameter"
equation "pcbOffset = 0.25 mm"
equation "wallThickness = 2 mm"
equation "d30 = pcbOffset"
equation "d31 = -pcbOffset"
equation "d32 = pcbOffset + wallThickness"
equation "pierDepth = 7 mm"
equation "pcbThickness = 1.6 mm"
equation "caseHeight = 22 mm"
equation "pierHeight = caseHeight - pcbThickness"
equation "pierBaseHeight = caseHeight - pierDepth - wallThickness"
equation "d38 = pierHeight"
equation "d40 = pierBaseHeight"
equation "d42 = pierBaseHeight"
equation "d44 = pierHeight"
equation "d46 = pierBaseHeight"
equation "d48 = pierHeight"
equation "d50 = pierBaseHeight"
equation "d52 = pierHeight"
equation "d54 = wallThickness"
equation "d56 = wallThickness"
equation "d58 = pierHeight"
equation "d60 = pierHeight"
equation "d62 = caseHeight"
equation "filletRadius = 1.5 mm"
equation "d66 = filletRadius"
equation "d68 = filletRadius"
equation "d70 = filletRadius"
equation "d72 = filletRadius"
equation "d74 = filletRadius"
equation "textThickness = 1.5 mm"
